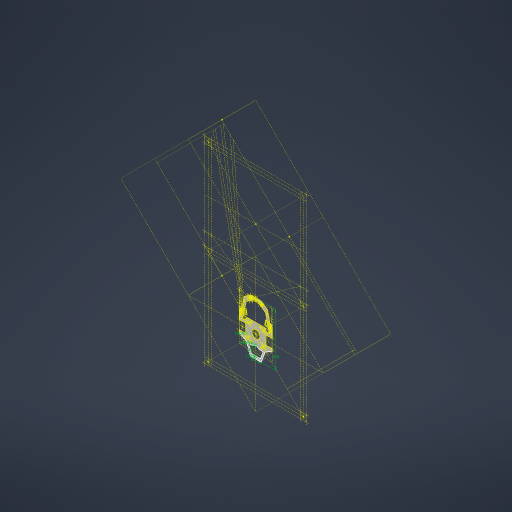
# Autodesk Inventor part: chassis-2
Saved by Autodesk Inventor 2023.5 (Build 275446000, 446)
## iProperties
Created: 2025-01-11
Part Number: chassis-2
Material: 一般
Document SubType Name: Modeling
Designer: IshiiLabHonda
Density: 1 g/cm^3
Appearance: 既定
Author: IshiiLabHonda
Autodesk Inventor part; units mm, degrees
ref_plane "YZ Plane" through (0, 0, 0) normal (1, 0, 0) x (0, 1, 0)
ref_plane "XZ Plane" through (0, 0, 0) normal (0, 1, 0) x (-1, 0, 0)
ref_plane "XY Plane" through (0, 0, 0) normal (0, 0, 1) x (1, 0, 0)
derived "chassis.ipt"
sketch "スケッチ1" plane through (0, 0, 0) normal (0, 0, 1) x (1, 0, 0)
  line L0 (0, 0) -> (0, 1) construction
  line L1 (0, 0) -> (1, 0) construction
  line L2 (-90, 90) -> (90, 90) construction
  line L3 (90, 90) -> (90, -90) construction
  line L4 (90, -90) -> (-90, -90) construction
  line L5 (-90, -90) -> (-90, 90) construction
  line L6 (-90, -90) -> (90, 90) construction
  line L7 (-90, 90) -> (90, -90) construction
  line L8 (-84, 96) -> (-84, 84) construction
  line L9 (-84, 84) -> (-96, 84) construction
  line L10 (-96, 84) -> (-96, 96) construction
  line L11 (-96, 96) -> (-84, 84) construction
  line L12 (-84, 96) -> (-96, 84) construction
  line L13 (-96, 96) -> (-84, 96) construction
  line L14 (-96, -96) -> (-96, -84) construction
  line L15 (-84, -96) -> (-96, -96) construction
  line L16 (-96, -96) -> (-84, -84) construction
  line L17 (-96, -84) -> (-84, -96) construction
  line L18 (-84, -84) -> (-84, -96) construction
  line L19 (-96, -84) -> (-84, -84) construction
  line L20 (96, -96) -> (84, -96) construction
  line L21 (96, -84) -> (96, -96) construction
  line L22 (96, -96) -> (84, -84) construction
  line L23 (84, -96) -> (96, -84) construction
  line L24 (84, -84) -> (96, -84) construction
  line L25 (84, -96) -> (84, -84) construction
  line L26 (96, 96) -> (96, 84) construction
  line L27 (84, 96) -> (96, 96) construction
  line L28 (96, 96) -> (84, 84) construction
  line L29 (96, 84) -> (84, 96) construction
  line L30 (84, 84) -> (84, 96) construction
  line L31 (96, 84) -> (84, 84) construction
  line L32 (-84, 84) -> (-84, -84) construction
  line L33 (-96, 84) -> (-96, -84) construction
  line L34 (-84, -84) -> (84, -84) construction
  line L35 (-84, -96) -> (84, -96) construction
  line L36 (96, 84) -> (96, -84) construction
  line L37 (84, 84) -> (84, -84) construction
  line L38 (-84, 96) -> (84, 96) construction
  line L39 (-84, 84) -> (84, 84) construction
  line L40 (-19, 15) -> (19, 15) construction
  line L41 (19, 15) -> (19, -15) construction
  line L42 (19, -15) -> (-19, -15) construction
  line L43 (-19, -15) -> (-19, 15) construction
  line L44 (-19, 15) -> (19, -15) construction
  line L45 (19, 15) -> (-19, -15) construction
  line L46 (-30.25, 11.5) -> (-19, 11.5) construction
  line L47 (-19, -11.5) -> (-30.25, -11.5) construction
  line L48 (-30.25, -11.5) -> (-30.25, 11.5) construction
  line L49 (-30.25, 11.5) -> (-19, -11.5) construction
  line L50 (-19, 11.5) -> (-30.25, -11.5) construction
  line L51 (19, 11.5) -> (30.25, -11.5) construction
  line L52 (19, -11.5) -> (30.25, -11.5) construction
  line L53 (30.25, -11.5) -> (30.25, 11.5) construction
  line L54 (30.25, 11.5) -> (19, 11.5) construction
  line L55 (30.25, 11.5) -> (19, -11.5) construction
  line L56 (-19, -10) -> (19, -10) construction
  line L57 (-19, -12.5) -> (19, -12.5) construction
  line L58 (-19, 12.5) -> (19, 12.5) construction
  line L59 (-19, 10) -> (19, 10) construction
  line L60 (-16.5, -15) -> (-16.5, 15) construction
  line L61 (16.5, -15) -> (16.5, 15) construction
  line L62 (-12.5, -10) -> (-12.5, -15) construction
  line L63 (-16.5, -10) -> (-12.5, -15) construction
  line L64 (-16.5, -15) -> (-12.5, -10) construction
  circle A0 centre (-14.5, -12.5) radius 0.8 construction
  line L65 (12.5, -10) -> (12.5, -15) construction
  line L66 (16.5, -10) -> (12.5, -15) construction
  circle A1 centre (14.5, -12.5) radius 0.8 construction
  line L67 (16.5, -15) -> (12.5, -10) construction
  line L68 (-12.5, 10) -> (-12.5, 15) construction
  line L69 (-16.5, 10) -> (-12.5, 15) construction
  line L70 (-16.5, 15) -> (-12.5, 10) construction
  circle A2 centre (-14.5, 12.5) radius 0.8 construction
  line L71 (12.5, 10) -> (12.5, 15) construction
  line L72 (16.5, 10) -> (12.5, 15) construction
  circle A3 centre (14.5, 12.5) radius 0.8 construction
  line L73 (16.5, 15) -> (12.5, 10) construction
  line L74 (-96, 276) -> (-84, 276) construction
  line L75 (-84, 276) -> (-84, 264) construction
  line L76 (-84, 264) -> (-96, 264) construction
  line L77 (-96, 264) -> (-96, 276) construction
  line L78 (-96, 276) -> (-84, 264) construction
  line L79 (-84, 276) -> (-96, 264) construction
  line L80 (-90, 90) -> (-90, 270) construction
  line L81 (-96, 264) -> (-96, 96) construction
  line L82 (-84, 264) -> (-84, 96) construction
  line L83 (84, 264) -> (84, 96) construction
  line L84 (90, 90) -> (90, 270) construction
  line L85 (96, 264) -> (96, 96) construction
  line L86 (84, 264) -> (96, 264) construction
  line L87 (84, 276) -> (84, 264) construction
  line L88 (96, 276) -> (84, 276) construction
  line L89 (96, 276) -> (84, 264) construction
  line L90 (84, 276) -> (96, 264) construction
  line L91 (96, 264) -> (96, 276) construction
  line L92 (-84, 276) -> (84, 276) construction
  line L93 (-84, 264) -> (84, 264) construction
  line L94 (-90, 270) -> (90, 270) construction
  line L95 (-90, 270) -> (90, 90) construction
  line L96 (-90, 90) -> (90, 270) construction
  circle A4 centre (0, 0) radius 15 construction
  line L97 (-96, 120) -> (96, 120) construction
  line L98 (0, 127.2792) -> (0, -127.2792) construction
  line L99 (-127.2792, 0) -> (127.2792, 0) construction
  line L100 (127.2792, 0) -> (0, -127.2792) construction
  line L101 (0, -127.2792) -> (-127.2792, 0) construction
  line L102 (-127.2792, 0) -> (0, 127.2792) construction
  line L103 (0, 127.2792) -> (127.2792, 0) construction
  line L104 (127.2792, 254.5584) -> (254.5584, 127.2792) construction
  line L105 (254.5584, 127.2792) -> (127.2792, 0) construction
  line L106 (127.2792, 0) -> (0, 127.2792) construction
  line L107 (0, 127.2792) -> (127.2792, 254.5584) construction
  line L108 (-127.2792, 254.5584) -> (0, 127.2792) construction
  line L109 (0, 127.2792) -> (-127.2792, 0) construction
  line L110 (-127.2792, 0) -> (-254.5584, 127.2792) construction
  line L111 (-254.5584, 127.2792) -> (-127.2792, 254.5584) construction
  line L112 (0, 381.8377) -> (127.2792, 254.5584) construction
  line L113 (127.2792, 254.5584) -> (0, 127.2792) construction
  line L114 (0, 127.2792) -> (-127.2792, 254.5584) construction
  line L115 (-127.2792, 254.5584) -> (0, 381.8377) construction
  line L116 (190.9188, 63.6396) -> (63.6396, 190.9188) construction
  line L117 (-190.9188, 190.9188) -> (-63.6396, 63.6396) construction
  line L118 (59.397, -59.397) -> (186.6762, 67.8823) construction
  line L119 (59.397, 186.6762) -> (186.6762, 59.397) construction
  line L120 (63.6396, 190.9188) -> (-63.6396, 318.1981) construction
  line L121 (-186.6762, 186.6762) -> (-59.397, 313.9554) construction
  point P0 (-90, -90)
  point P1 (90, -90)
  point P2 (-24.625, 0)
  point P3 (-84, 120)
  point P4 (84, 120)
  point P5 (0, 0)
sketch "スケッチ5" plane through (0, 0, 0) normal (0, 0, 1) x (1, 0, 0)
  line L0 (0, 0) -> (0, 1) construction
  line L1 (30.25, 11.5) -> (19, 11.5) construction
  line L2 (19, 11.5) -> (30.25, -11.5) construction
  line L3 (30.25, 11.5) -> (19, -11.5) construction
  line L4 (30.25, -11.5) -> (30.25, 11.5) construction
  line L5 (19, -11.5) -> (30.25, -11.5) construction
  line L6 (-90, 90) -> (90, 90) construction
  line L7 (-90, -90) -> (90, 90) construction
  line L8 (-90, 90) -> (90, -90) construction
  line L9 (-84, 84) -> (-84, -84) construction
  line L10 (-96, 84) -> (-96, -84) construction
  line L11 (-90, -90) -> (-90, 90) construction
  line L12 (-84, 84) -> (-96, 84) construction
  line L13 (-96, 84) -> (-96, 96) construction
  line L14 (84, 84) -> (84, -84) construction
  line L15 (90, 90) -> (90, -90) construction
  line L16 (96, 84) -> (84, 84) construction
  line L17 (96, 84) -> (96, -84) construction
  line L18 (90, -90) -> (-90, -90) construction
  line L19 (-84, -84) -> (84, -84) construction
  line L20 (-84, -96) -> (84, -96) construction
  line L21 (-84, -84) -> (-84, -96) construction
  line L22 (-96, -96) -> (-96, -84) construction
  line L23 (-84, -96) -> (-96, -96) construction
  line L24 (-96, -96) -> (-84, -84) construction
  line L25 (-96, -84) -> (-84, -96) construction
  line L26 (-96, -84) -> (-84, -84) construction
  line L27 (0, 0) -> (1, 0) construction
  line L28 (-84, 264) -> (-96, 264) construction
  line L29 (-96, 276) -> (-84, 276) construction
  line L30 (-96, 264) -> (-96, 276) construction
  line L31 (-84, 276) -> (-96, 264) construction
  line L32 (-96, 276) -> (-84, 264) construction
  line L33 (-84, 276) -> (-84, 264) construction
  line L34 (84, -96) -> (84, -84) construction
  line L35 (96, -96) -> (84, -96) construction
  line L36 (96, -84) -> (96, -96) construction
  line L37 (96, -96) -> (84, -84) construction
  line L38 (84, -96) -> (96, -84) construction
  line L39 (84, -84) -> (96, -84) construction
  line L40 (-19, 15) -> (19, 15) construction
  line L41 (19, 15) -> (19, -15) construction
  line L42 (16.5, 15) -> (12.5, 10) construction
  line L43 (12.5, 10) -> (12.5, 15) construction
  line L44 (16.5, 10) -> (12.5, 15) construction
  line L45 (16.5, -15) -> (16.5, 15) construction
  line L46 (-19, 10) -> (19, 10) construction
  line L47 (-19, 12.5) -> (19, 12.5) construction
  circle A0 centre (0, 0) radius 15 construction
  line L48 (-19, -10) -> (19, -10) construction
  line L49 (-19, -12.5) -> (19, -12.5) construction
  line L50 (19, -15) -> (-19, -15) construction
  line L51 (-19, 15) -> (19, -15) construction
  line L52 (19, 15) -> (-19, -15) construction
  line L53 (-16.5, -15) -> (-16.5, 15) construction
  line L54 (-19, -15) -> (-19, 15) construction
  line L55 (-30.25, 11.5) -> (-19, 11.5) construction
  line L56 (-19, -11.5) -> (-30.25, -11.5) construction
  line L57 (-30.25, -11.5) -> (-30.25, 11.5) construction
  line L58 (-30.25, 11.5) -> (-19, -11.5) construction
  line L59 (-19, 11.5) -> (-30.25, -11.5) construction
  line L60 (-12.5, 10) -> (-12.5, 15) construction
  circle A1 centre (-14.5, 12.5) radius 0.8 construction
  line L61 (-16.5, 10) -> (-12.5, 15) construction
  line L62 (-16.5, 15) -> (-12.5, 10) construction
  circle A2 centre (14.5, 12.5) radius 0.8 construction
  line L63 (-84, 96) -> (-96, 84) construction
  line L64 (-96, 96) -> (-84, 96) construction
  line L65 (-84, 96) -> (-84, 84) construction
  line L66 (-96, 96) -> (-84, 84) construction
  line L67 (-96, 264) -> (-96, 96) construction
  line L68 (-84, 264) -> (-84, 96) construction
  line L69 (-84, 96) -> (84, 96) construction
  line L70 (-84, 84) -> (84, 84) construction
  line L71 (84, 84) -> (84, 96) construction
  line L72 (96, 96) -> (96, 84) construction
  line L73 (96, 96) -> (84, 84) construction
  line L74 (96, 84) -> (84, 96) construction
  line L75 (-96, 120) -> (96, 120) construction
  line L76 (84, 96) -> (96, 96) construction
  line L77 (-84, 264) -> (84, 264) construction
  line L78 (84, 264) -> (84, 96) construction
  line L79 (-84, 276) -> (84, 276) construction
  line L80 (96, 264) -> (96, 96) construction
  line L81 (-90, 270) -> (90, 270) construction
  line L82 (-90, 270) -> (90, 90) construction
  line L83 (-90, 90) -> (90, 270) construction
  line L84 (90, 90) -> (90, 270) construction
  line L85 (-90, 90) -> (-90, 270) construction
  line L86 (84, 264) -> (96, 264) construction
  line L87 (96, 276) -> (84, 276) construction
  line L88 (96, 276) -> (84, 264) construction
  line L89 (84, 276) -> (96, 264) construction
  line L90 (96, 264) -> (96, 276) construction
  line L91 (84, 276) -> (84, 264) construction
  circle A3 centre (-14.5, -12.5) radius 0.8 construction
  line L92 (-12.5, -10) -> (-12.5, -15) construction
  line L93 (-16.5, -15) -> (-12.5, -10) construction
  line L94 (12.5, -10) -> (12.5, -15) construction
  circle A4 centre (14.5, -12.5) radius 0.8 construction
  line L95 (16.5, -15) -> (12.5, -10) construction
  line L96 (16.5, -10) -> (12.5, -15) construction
  line L97 (-16.5, -10) -> (-12.5, -15) construction
  line L98 (-12.9773, 53.9269) -> (-10.5199, 55.6476) construction
  line L99 (-8.7991, 53.1902) -> (-12.9773, 53.9269) construction
  circle A5 centre (-10.8882, 53.5585) radius 0.8 construction
  line L100 (-8.7991, 53.1902) -> (-11.2566, 51.4694) construction
  line L101 (-10.5199, 55.6476) -> (-11.2566, 51.4694) construction
  line L102 (-11.2566, 51.4694) -> (-12.9773, 53.9269) construction
  line L103 (-30.25, 44.8844) -> (-31, 44.3592) construction
  line L104 (-12.9471, 57) -> (-30.25, 44.8844) construction
  line L105 (-30.25, 57) -> (-31, 57) construction
  line L106 (-10.5199, 55.6476) -> (-8.7991, 53.1902) construction
  line L107 (-30.25, 57) -> (30.25, 57) construction
  line L108 (-6.2185, 52.5556) -> (-11.543, 48.8274) construction
  line L109 (-11.543, 48.8274) -> (-15.558, 54.5615) construction
  line L110 (-10.2335, 58.2897) -> (-6.2185, 52.5556) construction
  line L111 (1.0005, 57) -> (-30.25, 35.1182) construction
  line L112 (-1.0005, 57) -> (30.25, 35.1182) construction
  line L113 (-19, 15) -> (19, 15) construction
  line L114 (12.5, 10) -> (12.5, 15) construction
  line L115 (-19, 10) -> (19, 10) construction
  circle A6 centre (-14.5, 12.5) radius 0.8 construction
  line L116 (-12.5, 10) -> (-12.5, 15) construction
  line L117 (-16.5, 10) -> (-12.5, 15) construction
  line L118 (-16.5, 15) -> (-12.5, 10) construction
  line L119 (-19, 12.5) -> (19, 12.5) construction
  line L120 (30.25, 57) -> (31, 57) construction
  line L121 (30.25, 11.5) -> (30.25, 57) construction
  line L122 (-6.1403, 52) -> (6.1403, 52) construction
  line L123 (-30.25, 35.1182) -> (-31, 34.593) construction
  line L124 (-30.25, 11.5) -> (-30.25, 57) construction
  line L125 (-6.7921, 53.3748) -> (-12.1165, 49.6465) construction
  line L126 (-10.8882, 53.5585) -> (-10.4294, 52.9032) construction
  line L127 (-10.8882, 53.5585) -> (-10.2329, 54.0174) construction
  line L128 (-6.2185, 52.5556) -> (-15.558, 54.5615) construction
  line L129 (-9.6599, 57.4705) -> (-14.9844, 53.7423) construction
  line L130 (-15.558, 54.5615) -> (-10.2335, 58.2897) construction
  line L131 (-10.2335, 58.2897) -> (-11.543, 48.8274) construction
  line L132 (-30.25, 11.5) -> (-19, 11.5) construction
  line L133 (-30.25, 11.5) -> (-19, -11.5) construction
  line L134 (30.25, 11.5) -> (19, 11.5) construction
  line L135 (30.25, -11.5) -> (30.25, 11.5) construction
  line L136 (19, 11.5) -> (30.25, -11.5) construction
  line L137 (30.25, 11.5) -> (19, -11.5) construction
  line L138 (0, 0) -> (0, 1) construction
  line L139 (0, 0) -> (1, 0) construction
  circle A7 centre (0, 0) radius 7.5 construction
  circle A8 centre (0, 0) radius 15 construction
  line L140 (-16.5, -15) -> (-16.5, 15) construction
  circle A9 centre (14.5, 12.5) radius 0.8 construction
  line L141 (-12.5, -10) -> (-12.5, -15) construction
  line L142 (12.5, -10) -> (12.5, -15) construction
  line L143 (16.5, 10) -> (12.5, 15) construction
  line L144 (-16.5, -15) -> (-12.5, -10) construction
  line L145 (16.5, -10) -> (12.5, -15) construction
  line L146 (16.5, 15) -> (12.5, 10) construction
  line L147 (-19, -12.5) -> (19, -12.5) construction
  line L148 (19, -15) -> (-19, -15) construction
  line L149 (-19, 11.5) -> (-30.25, -11.5) construction
  line L150 (19, -11.5) -> (30.25, -11.5) construction
  line L151 (-19, -11.5) -> (-30.25, -11.5) construction
  line L152 (-30.25, -11.5) -> (-30.25, 11.5) construction
  line L153 (16.5, -15) -> (16.5, 15) construction
  line L154 (19, 15) -> (19, -15) construction
  line L155 (-19, -15) -> (-19, 15) construction
  line L156 (-19, 15) -> (19, -15) construction
  line L157 (19, 15) -> (-19, -15) construction
  line L158 (-31, -8.5) -> (31, -8.5) construction
  line L159 (-31, 8.5) -> (31, 8.5) construction
  line L160 (-31, -31) -> (31, -31) construction
  line L161 (-31, 57) -> (-31, -31) construction
  line L162 (31, 57) -> (31, -31) construction
  line L163 (84, -84) -> (96, -84) construction
  line L164 (84, -96) -> (96, -84) construction
  line L165 (96, -96) -> (84, -84) construction
  line L166 (96, -84) -> (96, -96) construction
  line L167 (96, -96) -> (84, -96) construction
  line L168 (-96, 84) -> (-96, -84) construction
  line L169 (-84, 84) -> (-84, -84) construction
  line L170 (-90, -90) -> (-90, 90) construction
  line L171 (-84, -84) -> (84, -84) construction
  line L172 (-84, -96) -> (84, -96) construction
  line L173 (-90, -90) -> (90, 90) construction
  line L174 (90, -90) -> (-90, -90) construction
  line L175 (-90, 90) -> (90, -90) construction
  line L176 (84, 84) -> (84, -84) construction
  line L177 (90, 90) -> (90, -90) construction
  line L178 (96, 84) -> (96, -84) construction
  line L179 (84, -96) -> (84, -84) construction
  line L180 (-19, -10) -> (19, -10) construction
  circle A10 centre (14.5, -12.5) radius 0.8 construction
  line L181 (16.5, -15) -> (12.5, -10) construction
  line L182 (-16.5, -10) -> (-12.5, -15) construction
  line L183 (-84, -84) -> (-84, -96) construction
  line L184 (-96, -84) -> (-84, -84) construction
  line L185 (-84, -96) -> (-96, -96) construction
  line L186 (-96, -96) -> (-84, -84) construction
  line L187 (-96, -84) -> (-84, -96) construction
  line L188 (-96, -96) -> (-96, -84) construction
  circle A11 centre (-14.5, -12.5) radius 0.8 construction
  line L189 (-96, 96) -> (-84, 96) construction
  line L190 (-84, 96) -> (-84, 84) construction
  line L191 (-84, 96) -> (-96, 84) construction
  line L192 (-96, 96) -> (-84, 84) construction
  line L193 (84, 96) -> (96, 96) construction
  line L194 (96, 84) -> (84, 84) construction
  line L195 (96, 96) -> (96, 84) construction
  line L196 (96, 96) -> (84, 84) construction
  line L197 (96, 84) -> (84, 96) construction
  line L198 (-96, 120) -> (96, 120) construction
  line L199 (-84, 96) -> (84, 96) construction
  line L200 (-90, 90) -> (90, 90) construction
  line L201 (-84, 84) -> (-96, 84) construction
  line L202 (-96, 84) -> (-96, 96) construction
  line L203 (-84, 84) -> (84, 84) construction
  line L204 (84, 120) -> (-30.25, 40.0013) construction
  line L205 (-84, 120) -> (30.25, 40.0013) construction
  line L206 (84, 84) -> (84, 96) construction
  line L207 (-84, 264) -> (-96, 264) construction
  line L208 (-90, 90) -> (-90, 270) construction
  line L209 (-96, 264) -> (-96, 96) construction
  line L210 (-84, 264) -> (-84, 96) construction
  line L211 (96, 264) -> (96, 96) construction
  line L212 (84, 264) -> (84, 96) construction
  line L213 (90, 90) -> (90, 270) construction
  line L214 (-90, 90) -> (90, 270) construction
  line L215 (-90, 270) -> (90, 90) construction
  line L216 (-84, 264) -> (84, 264) construction
  line L217 (-90, 270) -> (90, 270) construction
  line L218 (-96, 264) -> (-96, 276) construction
  line L219 (-96, 276) -> (-84, 276) construction
  line L220 (-96, 276) -> (-84, 264) construction
  line L221 (-84, 276) -> (-96, 264) construction
  line L222 (-84, 276) -> (-84, 264) construction
  line L223 (-84, 276) -> (84, 276) construction
  line L224 (84, 264) -> (96, 264) construction
  line L225 (96, 264) -> (96, 276) construction
  line L226 (96, 276) -> (84, 264) construction
  line L227 (96, 276) -> (84, 276) construction
  line L228 (84, 276) -> (96, 264) construction
  line L229 (84, 276) -> (84, 264) construction
  line L230 (-31, 8.5) -> (-19, 8.5) projected
  line L231 (-31, -8.5) -> (-19, -8.5) projected
  line L232 (-19, 8.5) -> (-19, -8.5) projected
  circle A12 centre (0, 0) radius 7.5 projected
  line L233 (31, -8.5) -> (19, -8.5) projected
  line L234 (19, 8.5) -> (19, -8.5) projected
  line L235 (31, 8.5) -> (19, 8.5) projected
  line L236 (31, 8.5) -> (31, 8.5) projected
  line L237 (-31, -8.5) -> (-12.1203, -31) construction
  line L238 (-12.1203, -31) -> (12.1203, -31) construction
  line L239 (31, -8.5) -> (12.1203, -31) construction
  circle A13 centre (-14.5, 12.5) radius 1.05 projected
  circle A14 centre (14.5, 12.5) radius 1.05 projected
  circle A15 centre (-14.5, -12.5) radius 1.05 projected
  circle A16 centre (14.5, -12.5) radius 1.05 projected
  line L240 (-26.25, 26.5) -> (-26.3613, 27.2922) construction
  line L241 (-26.25, 26.5) -> (-25.4578, 26.6113) construction
  circle A17 centre (-26.25, 26.5) radius 0.8 construction
  line L242 (-24.1223, 29.3236) -> (-23.4264, 24.3723) construction
  line L243 (-28.3777, 23.6764) -> (-29.0736, 28.6277) construction
  line L244 (-24.1223, 29.3236) -> (-28.3777, 23.6764) construction
  line L245 (-29.0736, 28.6277) -> (-24.1223, 29.3236) construction
  line L246 (-23.4264, 24.3723) -> (-28.3777, 23.6764) construction
  line L247 (-29.0736, 28.6277) -> (-23.4264, 24.3723) construction
  line L248 (-29.0736, 28.6277) -> (-28.3777, 23.6764) projected
  line L249 (-24.1223, 29.3236) -> (-19.1709, 30.0195) construction
  line L250 (-19.1709, 30.0195) -> (-18.4751, 25.0681) construction
  line L251 (-18.4751, 25.0681) -> (-23.4264, 24.3723) construction
  line L252 (28.3777, 23.6764) -> (23.4264, 24.3723) construction
  line L253 (18.4751, 25.0681) -> (23.4264, 24.3723) construction
  line L254 (19.1709, 30.0195) -> (18.4751, 25.0681) construction
  line L255 (24.1223, 29.3236) -> (19.1709, 30.0195) construction
  line L256 (24.1223, 29.3236) -> (29.0736, 28.6277) construction
  line L257 (29.0736, 28.6277) -> (28.3777, 23.6764) construction
  line L258 (-29.0736, 28.6277) -> (-19.1709, 30.0195) projected
  line L259 (-18.4751, 25.0681) -> (-19.1709, 30.0195) projected
  line L260 (-18.4751, 25.0681) -> (-28.3777, 23.6764) projected
  line L261 (19.1709, 30.0195) -> (29.0736, 28.6277) projected
  line L262 (28.3777, 23.6764) -> (29.0736, 28.6277) projected
  line L263 (28.3777, 23.6764) -> (18.4751, 25.0681) projected
  line L264 (19.1709, 30.0195) -> (18.4751, 25.0681) projected
  line L265 (-9.6771, 59.2897) -> (9.6771, 59.2897) projected
  line L266 (-9.6771, 59.2897) -> (-9.6771, 59.2897) projected
  line L267 (-3.6771, 59.2897) -> (-0.9296, 58.2897) projected
  line L268 (-0.9296, 58.2897) -> (0.9296, 58.2897) projected
  line L269 (0.9296, 58.2897) -> (3.6771, 59.2897) projected
  line L270 (-4.6137, 54.2897) -> (4.6137, 54.2897) projected
  line L271 (-18.1736, 44.795) -> (-4.6137, 54.2897) projected
  line L272 (-31, 8.5) -> (-22.0451, 50.6295) projected
  line L273 (-22.0451, 50.6295) -> (-9.6771, 59.2897) projected
  line L274 (31, 8.5) -> (22.0451, 50.6295) projected
  line L275 (-18.1736, 44.795) -> (-23.6565, 19) projected
  line L276 (18.1736, 44.795) -> (23.6565, 19) projected
  line L277 (-23.6565, 19) -> (23.6565, 19) projected
  line L278 (-17.6308, -20) -> (17.6308, -20) construction
  line L279 (17.6308, -20) -> (11.5077, -26) construction
  line L280 (11.5077, -26) -> (-11.5077, -26) construction
  line L281 (-11.5077, -26) -> (-17.6308, -20) construction
  line L282 (-31, -8.5) -> (-31, -12.5) projected
  line L283 (-31, -12.5) -> (-12.1203, -31) construction
  line L284 (31, -8.5) -> (31, -12.5) projected
  line L285 (31, -12.5) -> (12.1203, -31) construction
  line L286 (-31, 8.5) -> (-31, 26.5) projected
  line L287 (-31, 26.5) -> (-26.3435, 30.4073) projected
  line L288 (31, 26.5) -> (26.3435, 30.4073) projected
  line L289 (31, 8.5) -> (31, 26.5) projected
  line L290 (-8.1203, -31) -> (-6.6203, -29.5) construction
  line L291 (-6.6203, -29.5) -> (6.6203, -29.5) construction
  line L292 (6.6203, -29.5) -> (8.1203, -31) construction
  line L293 (22.0451, 50.6295) -> (9.6771, 59.2897) projected
  line L294 (18.1736, 44.795) -> (4.6137, 54.2897) projected
  line L295 (-23.6565, 19) -> (-24.8255, 13.5) projected
  line L296 (-24.8255, 13.5) -> (-20.8255, 13.5) projected
  line L297 (-20.8255, 13.5) -> (-15.3255, 19) projected
  line L298 (23.6565, 19) -> (24.8255, 13.5) projected
  line L299 (24.8255, 13.5) -> (20.8255, 13.5) projected
  line L300 (20.8255, 13.5) -> (15.3255, 19) projected
  line L301 (-17.6308, -20) -> (-24.2643, -13.5) construction
  line L302 (-24.2643, -13.5) -> (-21.2643, -13.5) construction
  line L303 (-21.2643, -13.5) -> (-11.6308, -20) construction
  line L304 (21.2643, -13.5) -> (11.6308, -20) construction
  line L305 (17.6308, -20) -> (24.2643, -13.5) construction
  line L306 (24.2643, -13.5) -> (21.2643, -13.5) construction
  circle A18 centre (-10.1308, -17) radius 0.625 construction
  circle A19 centre (-10.1308, -17) radius 0.8 projected
  circle A20 centre (-10.1308, -17) radius 1.5 projected
  line L307 (-11.6308, -20) -> (-11.6308, -15) construction
  circle A21 centre (10.1308, -17) radius 0.625 construction
  circle A22 centre (10.1308, -17) radius 0.8 projected
  circle A23 centre (10.1308, -17) radius 1.5 projected
  circle A24 centre (-9, 15.5) radius 0.625 construction
  circle A25 centre (-9, 15.5) radius 0.8 projected
  circle A26 centre (-9, 15.5) radius 1.5 projected
  circle A27 centre (9, 15.5) radius 0.625 construction
  circle A28 centre (9, 15.5) radius 0.8 projected
  circle A29 centre (9, 15.5) radius 1.5 projected
  circle A30 centre (-21.0348, 43.3585) radius 0.8 projected
  circle A31 centre (-21.0348, 43.3585) radius 1.5 construction
  circle A32 centre (21.0348, 43.3585) radius 0.8 projected
  circle A33 centre (21.0348, 43.3585) radius 1.5 construction
  circle A34 centre (21.0348, 43.3585) radius 0.475 construction
  line L308 (-30.8721, 30.6471) -> (-17.9987, 32.4563) projected
  line L309 (-17.9987, 32.4563) -> (-16.6765, 23.0488) projected
  line L310 (-16.6765, 23.0488) -> (-29.55, 21.2395) projected
  line L311 (-29.55, 21.2395) -> (-30.8721, 30.6471) projected
  line L312 (-22.0451, 50.6295) -> (-18.1736, 44.795) construction
  line L313 (-21.8107, 27.6837) -> (-26, 24.1685) projected
  line L314 (-26, 24.1685) -> (-26, 13.5) projected
  line L315 (-24.8255, 13.5) -> (-26, 13.5) projected
  line L316 (21.8107, 27.6837) -> (26, 24.1685) projected
  line L317 (26, 24.1685) -> (26, 13.5) projected
  line L318 (24.8255, 13.5) -> (26, 13.5) projected
  circle A35 centre (-28.5, 18.5) radius 0.8 projected
  circle A36 centre (-28.5, 18.5) radius 1.5 projected
  circle A37 centre (-28.5, 18.5) radius 0.475 construction
  circle A38 centre (28.5, 18.5) radius 0.475 construction
  circle A39 centre (28.5, 18.5) radius 0.8 projected
  circle A40 centre (28.5, 18.5) radius 1.5 projected
  line L319 (-12.9471, 57) -> (12.9471, 57) projected
  line L320 (30.8721, 30.6471) -> (17.9987, 32.4563) projected
  line L321 (17.9987, 32.4563) -> (16.6765, 23.0488) projected
  line L322 (16.6765, 23.0488) -> (29.55, 21.2395) projected
  line L323 (29.55, 21.2395) -> (30.8721, 30.6471) projected
  line L324 (-31, -12.5) -> (-10, -40.7103) construction
  line L325 (-10, -40.7103) -> (10, -40.7103)
  line L326 (10, -40.7103) -> (31, -12.5) construction
  line L327 (-31, -12.5) -> (-17.4124, -20.3448)
  line L328 (-17.4124, -20.3448) -> (-10, -40.7103)
  line L329 (31, -12.5) -> (17.4124, -20.3448)
  line L330 (17.4124, -20.3448) -> (10, -40.7103)
  line L331 (-7, -40.7103) -> (-5, -38.7103)
  line L332 (-5, -38.7103) -> (5, -38.7103)
  line L333 (5, -38.7103) -> (7, -40.7103)
  line L334 (-13.7229, -21.7103) -> (-8.6273, -35.7103)
  line L335 (-8.6273, -35.7103) -> (8.6273, -35.7103)
  line L336 (8.6273, -35.7103) -> (13.7229, -21.7103)
  line L337 (-6.2229, -21.7103) -> (-3, -18.7103)
  line L338 (-3, -18.7103) -> (3, -18.7103)
  line L339 (3, -18.7103) -> (6.2229, -21.7103)
  line L340 (-13.7229, -21.7103) -> (-6.2229, -21.7103)
  line L341 (6.2229, -21.7103) -> (13.7229, -21.7103)
  line L342 (-23.4801, 43.8782) -> (-18.5894, 42.8387) construction
  line L343 (-20.1093, 47.7123) -> (-28.4441, 8.5) construction
  line L344 (-13.2559, 53.976) -> (-10.4708, 55.9262) projected
  line L345 (-10.4708, 55.9262) -> (-8.5206, 53.1411) projected
  line L346 (-8.5206, 53.1411) -> (-11.3057, 51.1909) projected
  line L347 (-11.3057, 51.1909) -> (-13.2559, 53.976) projected
  line L348 (-13.2559, 53.976) -> (-8.5206, 53.1411) construction
  line L349 (-10.4708, 55.9262) -> (-11.3057, 51.1909) construction
  line L350 (13.2559, 53.976) -> (10.4708, 55.9262) projected
  line L351 (11.3057, 51.1909) -> (13.2559, 53.976) projected
  line L352 (8.5206, 53.1411) -> (11.3057, 51.1909) projected
  line L353 (10.4708, 55.9262) -> (8.5206, 53.1411) projected
  circle A41 centre (-10.8882, 53.5585) radius 1.05 projected
  circle A42 centre (10.8882, 53.5585) radius 1.05 projected
  point P0 (-90, -90)
  point P1 (90, -90)
  point P2 (-24.625, 0)
  point P3 (-8.226, 55.4227)
  point P4 (-5.9733, 57)
  point P5 (0, 61.1826)
  point P6 (-24.625, 0)
  point P7 (-90, -90)
  point P8 (90, -90)
  point P9 (-5.9733, 57)
  point P10 (5.9733, 57)
  point P11 (12.9773, 53.9269)
  point P12 (8.7991, 53.1902)
  point P13 (-15.4776, -12.7103)
  point P14 (-13.5224, -12.7103)
  point P15 (13.5224, -12.7103)
  point P16 (15.4776, -12.7103)
  dimension "d1" = 3
  dimension "d2" = 3
  dimension "d3" = 120
  dimension "d5" = 3
  dimension "d6" = 17
  dimension "d7" = 10
  dimension "d8" = 2
  dimension "d9" = 135
  dimension "d10" = 20
  dimension "d11" = 140
  dimension "d12" = 6
  dimension "d13" = 7.5
  dimension "d14" = 100
  constraints: 36 end point, 6 parallel, 5 horizontal alignment, 2 point on line, 1 perpendicular, 33 other
  measures "d1" distance between parallel lines of L332 L335
  measures "d2" distance between parallel lines of L328 L334
  measures "d3" angle of L327 L161
  measures "d5" distance between parallel lines of L340 L338
  measures "d6" distance between parallel lines of L335 L338
  measures "d7" distance of L331.end L332.end
  measures "d8" distance between parallel lines of L325 L332
  measures "d9" angle of L325 L331
  measures "d10" distance of L324.end L325.end
  measures "d11" angle of L328 L327
  measures "d12" distance of L337.end L338.end
  measures "d13" distance of L334.start L337.start
  measures "d14" distance between parallel lines of L325 L265
extrude "押し出し1" add sketch "スケッチ5" against normal blind 1 contours L272 A36 L310 L314 L315 L296 L297 L277 L300 L299 L318 L317 L322 L274 A40 L235 L234 L233 L284 L329 L330 L325 L333 L332 L331 L328 L327 L282 L231 L232 L230 | L286 L287 L311 L310 L272 A36 | L287 L248 L260 L272 L310 L311 | L272 L260 L314 L310 | L287 L258 L272 L260 L248 | L272 L258 L275 L313 L314 L260 | L314 L260 L275 L310 | L310 L275 L295 L315 L314 | L287 L272 L258 | L308 L275 L258 L272 | L272 L273 L319 L293 L274 L320 L276 L294 L270 L271 L275 L308 | L314 L313 L275 L260 | L273 L265 L267 L268 L269 L293 L319 | L276 L322 L317 L318 L298 | L274 L261 L276 L320 | L276 L263 L317 L322 | L288 L261 L274 | L276 L316 L317 L263 | L317 L263 L274 L322 | L274 L263 L317 L316 L276 L261 | L261 L288 L262 L263 L274 | L323 L322 L274 L263 L262 L288 | L288 L289 L274 A40 L322 L323 | A15 | A16 | A19 | A20 | A22 | A23 | A26 | A29 | L340 L337 L338 L339 L341 L336 L335 L334 | L344 L345 L346 L347 | L351 L352 L353 L350 | A41 | A42
extrude "押し出し2" cut sketch "スケッチ5" against normal blind 1.5 contours A15 | A16 | A19 | A22 | L340 L337 L338 L339 L341 L336 L335 L334
fillet "フィレット1" radius 2 4 edges at (-19, -8.5, -0.5) (-19, 8.5, -0.5) (19, 8.5, -0.5) (19, -8.5, -0.5)
chamfer "面取り1" distance 2 angle 45 2 edges at (-24.8255, 13.5, -0.5) (24.8255, 13.5, -0.5)
fillet "フィレット2" radius 0.8 26 edges at (-10, -40.7103, -0.5) (-7, -40.7103, -0.5) (-5, -38.7103, -0.5) (5, -38.7103, -0.5) (7, -40.7103, -0.5) (10, -40.7103, -0.5) (17.4124, -20.3448, -0.5) (31, -12.5, -0.5) (31, -8.5, -0.5) (31, 8.5, -0.5) (31, 26.5, -0.5) (26.3435, 30.4073, -0.5) (22.0451, 50.6295, -0.5) (9.6771, 59.2897, -0.5) (3.6771, 59.2897, -0.5) (0.9296, 58.2897, -0.5) (-0.9296, 58.2897, -0.5) (-3.6771, 59.2897, -0.5) (-9.6771, 59.2897, -0.5) (-22.0451, 50.6295, -0.5) (-26.3435, 30.4073, -0.5) (-31, 26.5, -0.5) (-31, 8.5, -0.5) (-31, -8.5, -0.5) (-31, -12.5, -0.5) (-17.4124, -20.3448, -0.5)
fillet "フィレット3" radius 0.8 20 edges at (-22.8255, 13.5, -0.5) (-20.8255, 13.5, -0.5) (-15.3255, 19, -0.5) (15.3255, 19, -0.5) (20.8255, 13.5, -0.5) (22.8255, 13.5, -0.5) (24.4097, 15.4563, -0.5) (18.1736, 44.795, -0.5) (4.6137, 54.2897, -0.5) (-4.6137, 54.2897, -0.5) (-18.1736, 44.795, -0.5) (-24.4097, 15.4563, -0.5) (-13.7229, -21.7103, -0.5) (-6.2229, -21.7103, -0.5) (-3, -18.7103, -0.5) (3, -18.7103, -0.5) (6.2229, -21.7103, -0.5) (13.7229, -21.7103, -0.5) (8.6273, -35.7103, -0.5) (-8.6273, -35.7103, -0.5)
extrude "押し出し3" cut sketch "スケッチ5" against normal blind 1 contours A41 | A42
sketch "スケッチ4" plane through (0, 0, 0) normal (0, 0, 1) x (1, 0, 0)
  line L0 (-84, 264) -> (-96, 264) construction
  line L1 (-90, 90) -> (-90, 270) construction
  line L2 (-96, 264) -> (-96, 96) construction
  line L3 (-96, 96) -> (-84, 96) construction
  line L4 (-84, 96) -> (-84, 84) construction
  line L5 (-84, 96) -> (-96, 84) construction
  line L6 (-96, 96) -> (-84, 84) construction
  line L7 (-84, 264) -> (-84, 96) construction
  line L8 (-84, 84) -> (-96, 84) construction
  line L9 (84, -84) -> (96, -84) construction
  line L10 (84, -96) -> (96, -84) construction
  line L11 (96, -96) -> (84, -84) construction
  line L12 (96, -84) -> (96, -96) construction
  line L13 (96, -96) -> (84, -96) construction
  line L14 (0, 0) -> (0, 1) construction
  line L15 (0, 0) -> (1, 0) construction
  line L16 (16.5, 15) -> (12.5, 10) construction
  line L17 (-96, 84) -> (-96, -84) construction
  line L18 (-84, 84) -> (-84, -84) construction
  line L19 (-90, -90) -> (-90, 90) construction
  line L20 (-90, 90) -> (90, 90) construction
  line L21 (-84, -84) -> (84, -84) construction
  line L22 (-84, -96) -> (84, -96) construction
  line L23 (-90, -90) -> (90, 90) construction
  line L24 (90, -90) -> (-90, -90) construction
  line L25 (-90, 90) -> (90, -90) construction
  line L26 (84, 84) -> (84, -84) construction
  line L27 (90, 90) -> (90, -90) construction
  line L28 (96, 84) -> (96, -84) construction
  line L29 (-96, 84) -> (-96, 96) construction
  line L30 (-84, -84) -> (-84, -96) construction
  line L31 (-96, -84) -> (-84, -84) construction
  line L32 (-84, -96) -> (-96, -96) construction
  line L33 (-96, -96) -> (-84, -84) construction
  line L34 (-96, -84) -> (-84, -96) construction
  line L35 (-96, -96) -> (-96, -84) construction
  line L36 (84, -96) -> (84, -84) construction
  line L37 (-19, -15) -> (-19, 15) construction
  line L38 (-30.25, 11.5) -> (-19, 11.5) construction
  line L39 (-19, -11.5) -> (-30.25, -11.5) construction
  line L40 (-19, 11.5) -> (-30.25, -11.5) construction
  line L41 (-30.25, 11.5) -> (-19, -11.5) construction
  line L42 (-30.25, -11.5) -> (-30.25, 11.5) construction
  line L43 (12.5, 10) -> (12.5, 15) construction
  circle A0 centre (14.5, 12.5) radius 0.8 construction
  line L44 (30.25, 11.5) -> (19, 11.5) construction
  line L45 (16.5, 10) -> (12.5, 15) construction
  circle A1 centre (14.5, -12.5) radius 0.8 construction
  line L46 (16.5, -15) -> (12.5, -10) construction
  line L47 (16.5, -10) -> (12.5, -15) construction
  line L48 (12.5, -10) -> (12.5, -15) construction
  circle A2 centre (-14.5, -12.5) radius 0.8 construction
  line L49 (-12.5, -10) -> (-12.5, -15) construction
  line L50 (-16.5, -15) -> (-12.5, -10) construction
  line L51 (-16.5, -10) -> (-12.5, -15) construction
  line L52 (96, 84) -> (84, 84) construction
  line L53 (96, 96) -> (96, 84) construction
  line L54 (84, 96) -> (96, 96) construction
  line L55 (96, 96) -> (84, 84) construction
  line L56 (84, 84) -> (84, 96) construction
  line L57 (96, 84) -> (84, 96) construction
  line L58 (-96, 264) -> (-96, 276) construction
  line L59 (-84, 276) -> (-84, 264) construction
  line L60 (-96, 276) -> (-84, 276) construction
  line L61 (-96, 276) -> (-84, 264) construction
  line L62 (-84, 276) -> (-96, 264) construction
  line L63 (-84, 84) -> (84, 84) construction
  line L64 (-84, 96) -> (84, 96) construction
  line L65 (84, 264) -> (84, 96) construction
  line L66 (90, 90) -> (90, 270) construction
  line L67 (-90, 90) -> (90, 270) construction
  line L68 (-90, 270) -> (90, 90) construction
  line L69 (96, 264) -> (96, 96) construction
  line L70 (-96, 120) -> (96, 120) construction
  line L71 (-84, 264) -> (84, 264) construction
  line L72 (-84, 276) -> (84, 276) construction
  line L73 (-90, 270) -> (90, 270) construction
  line L74 (84, 276) -> (84, 264) construction
  line L75 (84, 264) -> (96, 264) construction
  line L76 (96, 264) -> (96, 276) construction
  line L77 (96, 276) -> (84, 264) construction
  line L78 (96, 276) -> (84, 276) construction
  line L79 (84, 276) -> (96, 264) construction
  line L80 (-19, 15) -> (19, 15) construction
  line L81 (19, 15) -> (19, -15) construction
  line L82 (19, -15) -> (-19, -15) construction
  circle A3 centre (-14.5, 12.5) radius 0.8 construction
  line L83 (-16.5, 10) -> (-12.5, 15) construction
  line L84 (-12.5, 10) -> (-12.5, 15) construction
  line L85 (-16.5, 15) -> (-12.5, 10) construction
  circle A4 centre (0, 0) radius 15 construction
  line L86 (-19, 10) -> (19, 10) construction
  line L87 (-19, 12.5) -> (19, 12.5) construction
  line L88 (-19, 15) -> (19, -15) construction
  line L89 (19, 15) -> (-19, -15) construction
  line L90 (-19, -10) -> (19, -10) construction
  line L91 (-19, -12.5) -> (19, -12.5) construction
  line L92 (16.5, -15) -> (16.5, 15) construction
  line L93 (19, 11.5) -> (30.25, -11.5) construction
  line L94 (19, -11.5) -> (30.25, -11.5) construction
  line L95 (30.25, -11.5) -> (30.25, 11.5) construction
  line L96 (30.25, 11.5) -> (19, -11.5) construction
  line L97 (-16.5, -15) -> (-16.5, 15) construction
  line L98 (-84, 120) -> (30.25, 40.0013) construction
  line L99 (84, 120) -> (-30.25, 40.0013) construction
  line L100 (-30.25, 57) -> (30.25, 57) construction
  line L101 (1.0005, 57) -> (-30.25, 35.1182) construction
  line L102 (-1.0005, 57) -> (30.25, 35.1182) construction
  line L103 (-12.9471, 57) -> (-30.25, 44.8844) construction
  line L104 (-10.2335, 58.2897) -> (-6.2185, 52.5556) construction
  line L105 (-6.2185, 52.5556) -> (-11.543, 48.8274) construction
  line L106 (-11.543, 48.8274) -> (-15.558, 54.5615) construction
  line L107 (-15.558, 54.5615) -> (-10.2335, 58.2897) construction
  line L108 (-10.2335, 58.2897) -> (-11.543, 48.8274) construction
  line L109 (-6.2185, 52.5556) -> (-15.558, 54.5615) construction
  line L110 (-9.6599, 57.4705) -> (-14.9844, 53.7423) construction
  line L111 (-6.7921, 53.3748) -> (-12.1165, 49.6465) construction
  line L112 (-10.8882, 53.5585) -> (-10.2329, 54.0174) construction
  line L113 (-10.8882, 53.5585) -> (-10.4294, 52.9032) construction
  line L114 (-10.5199, 55.6476) -> (-8.7991, 53.1902) construction
  line L115 (-8.7991, 53.1902) -> (-11.2566, 51.4694) construction
  line L116 (-11.2566, 51.4694) -> (-12.9773, 53.9269) construction
  line L117 (-12.9773, 53.9269) -> (-10.5199, 55.6476) construction
  line L118 (-10.5199, 55.6476) -> (-11.2566, 51.4694) construction
  line L119 (-8.7991, 53.1902) -> (-12.9773, 53.9269) construction
  circle A5 centre (-10.8882, 53.5585) radius 0.8 construction
  line L120 (-30.25, 11.5) -> (-30.25, 57) construction
  line L121 (30.25, 11.5) -> (30.25, 57) construction
  line L122 (-6.1403, 52) -> (6.1403, 52) construction
  line L123 (-31, 57) -> (-31, -31) construction
  line L124 (31, 57) -> (31, -31) construction
  line L125 (-30.25, 57) -> (-31, 57) construction
  line L126 (30.25, 57) -> (31, 57) construction
  line L127 (-31, 8.5) -> (31, 8.5) construction
  line L128 (-31, -8.5) -> (31, -8.5) construction
  circle A6 centre (0, 0) radius 7.5 construction
  line L129 (-31, -31) -> (31, -31) construction
  line L130 (-30.25, 44.8844) -> (-31, 44.3592) construction
  line L131 (-30.25, 35.1182) -> (-31, 34.593) construction
  line L132 (-26.25, 26.5) -> (-26.3613, 27.2922) construction
  line L133 (-26.25, 26.5) -> (-25.4578, 26.6113) construction
  line L134 (-29.0736, 28.6277) -> (-24.1223, 29.3236) construction
  line L135 (-24.1223, 29.3236) -> (-23.4264, 24.3723) construction
  line L136 (-23.4264, 24.3723) -> (-28.3777, 23.6764) construction
  line L137 (-28.3777, 23.6764) -> (-29.0736, 28.6277) construction
  line L138 (-29.0736, 28.6277) -> (-23.4264, 24.3723) construction
  line L139 (-24.1223, 29.3236) -> (-28.3777, 23.6764) construction
  circle A7 centre (-26.25, 26.5) radius 0.8 construction
  line L140 (-26.25, 57) -> (-26.25, -31) construction
  line L141 (-96, 180) -> (96, 180) construction
  line L142 (-26.3613, 27.2922) -> (-65.7556, 307.5968) construction
  line L143 (-186.6762, 186.6762) -> (-59.397, 313.9554) construction
  line L144 (59.397, 186.6762) -> (186.6762, 59.397) construction
  line L145 (-26.25, 26.5) -> (-80.4501, 292.9022) construction
  line L146 (-26.25, 26.5) -> (-47.9742, 302.5327) construction
  line L147 (63.6396, 190.9188) -> (-63.6396, 318.1981) construction
  line L148 (10.8882, 53.5585) -> (10.2329, 54.0174) construction
  line L149 (10.8882, 53.5585) -> (10.4294, 52.9032) construction
  circle A8 centre (10.8882, 53.5585) radius 0.8 construction
  line L150 (12.9773, 53.9269) -> (10.5199, 55.6476) construction
  line L151 (10.5199, 55.6476) -> (11.2566, 51.4694) construction
  line L152 (11.2566, 51.4694) -> (12.9773, 53.9269) construction
  line L153 (11.543, 48.8274) -> (15.558, 54.5615) construction
  line L154 (8.7991, 53.1902) -> (11.2566, 51.4694) construction
  line L155 (6.7921, 53.3748) -> (12.1165, 49.6465) construction
  line L156 (10.5199, 55.6476) -> (8.7991, 53.1902) construction
  line L157 (6.2185, 52.5556) -> (15.558, 54.5615) construction
  line L158 (9.6599, 57.4705) -> (14.9844, 53.7423) construction
  line L159 (8.7991, 53.1902) -> (12.9773, 53.9269) construction
  line L160 (6.2185, 52.5556) -> (11.543, 48.8274) construction
  line L161 (10.2335, 58.2897) -> (6.2185, 52.5556) construction
  line L162 (15.558, 54.5615) -> (10.2335, 58.2897) construction
  line L163 (10.2335, 58.2897) -> (11.543, 48.8274) construction
  line L164 (-24.1223, 29.3236) -> (-19.1709, 30.0195) construction
  line L165 (-19.1709, 30.0195) -> (-18.4751, 25.0681) construction
  line L166 (-18.4751, 25.0681) -> (-23.4264, 24.3723) construction
  line L167 (-24.1223, 29.3236) -> (-29.0736, 28.6277) construction
  line L168 (-29.0736, 28.6277) -> (-28.3777, 23.6764) construction
  line L169 (-28.3777, 23.6764) -> (-23.4264, 24.3723) construction
  line L170 (24.1223, 29.3236) -> (29.0736, 28.6277) construction
  line L171 (28.3777, 23.6764) -> (23.4264, 24.3723) construction
  line L172 (18.4751, 25.0681) -> (23.4264, 24.3723) construction
  line L173 (28.3777, 23.6764) -> (29.0736, 28.6277) construction
  line L174 (19.1709, 30.0195) -> (18.4751, 25.0681) construction
  line L175 (24.1223, 29.3236) -> (19.1709, 30.0195) construction
  line L176 (29.0736, 28.6277) -> (28.3777, 23.6764) construction
  line L177 (24.1223, 29.3236) -> (28.3777, 23.6764) construction
  line L178 (23.4264, 24.3723) -> (29.0736, 28.6277) construction
  line L179 (-21.2987, 27.1959) -> (-61.3286, 312.0238) construction
  line L180 (-21.2987, 27.1959) -> (-42.5405, 297.0989) construction
  line L181 (-21.2987, 27.1959) -> (-76.2182, 297.1342) construction
  line L182 (-24.1223, 29.3236) -> (-18.4751, 25.0681) construction
  line L183 (-23.4264, 24.3723) -> (-19.1709, 30.0195) construction
  line L184 (-15.558, 54.5615) -> (-18.0155, 52.8407) construction
  line L185 (-18.0155, 52.8407) -> (-14.0004, 47.1067) construction
  line L186 (-14.0004, 47.1067) -> (-11.543, 48.8274) construction
  point P0 (90, -90)
  point P1 (-90, -90)
  point P2 (-24.625, 0)
  point P3 (0, 61.1826)
  point P4 (-5.9733, 57)
  point P5 (-8.226, 55.4227)
  point P6 (0, 180)
  point P7 (8.226, 55.4227)
  constraints: 2 other
